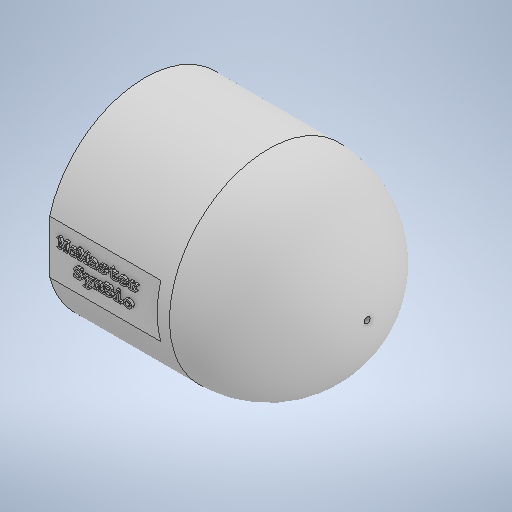
# Autodesk Inventor part: Bactria Membrane Half 1
Saved by Autodesk Inventor 2025 (Build 290162000, 162)
## iProperties
Created: 2024-08-12
Part Number: Bactria Membrane Half 1
Material: Generic
Document SubType Name: Modeling
Designer: kellst1
Density: 1 g/cm^3
Appearance: Default
Author: kellst1
Autodesk Inventor part; units mm, degrees
(part 1 of 2)
ref_plane "YZ Plane" through (0, 0, 0) normal (1, 0, 0) x (0, 1, 0)
ref_plane "XZ Plane" through (0, 0, 0) normal (0, 1, 0) x (-1, 0, 0)
ref_plane "XY Plane" through (0, 0, 0) normal (0, 0, 1) x (1, 0, 0)
sketch "Sketch1" plane through (0, 0, 0) normal (1, 0, 0) x (0, 1, 0)
  arc A0 (0, -80) -> (0, 80) centre (0, 0) ccw
  arc A1 (0, -65) -> (0, 65) centre (0, 0) ccw
  line L0 (0, 80) -> (0, -80)
  dimension "d0" = 160
  dimension "d1" = 130
  constraints: 4 point on circle, 2 centre point, 2 coincident, 2 end point, 2 point on line, 1 vertical
  measures "d0" diameter of A0
  measures "d1" diameter of A1
revolve "Revolution1" add sketch "Sketch1" angle 180 about axis through (0, 0, 80) along (0, 0, -1) contours L0 A1 A0
sketch "Sketch3" plane through (0, 0, 0) normal (-1, 0, 0) x (0, 0, 1)
  circle A0 centre (0, 0) radius 65
  circle A1 centre (0, 0) radius 80
  constraints: 2 centre point, 2 coincident
extrude "Extrusion2" add sketch "Sketch3" along normal blind 80
sketch "Sketch4" plane through (-80, 0, 0) normal (-1, 0, 0) x (0, 0, 1)
  circle A0 centre (0, 0) radius 72.5
  circle A1 centre (0, 0) radius 80
  dimension "d9" = 145
  dimension "d10" = 160
  constraints: 2 centre point, 1 coincident
  measures "d9" diameter of A0
  measures "d10" diameter of A1
extrude "Extrusion3" add sketch "Sketch4" along normal blind 20
thread "Thread2" size "M50x4" class "6H" standard "ANSI Metric M Profile" length 20
sketch "Sketch5" plane through (-100, 0, 0) normal (-1, 0, 0) x (0, 0, 1)
  circle A0 centre (0, 0) radius 2.5
  dimension "d15" = 5
  constraints: 1 centre point, 1 coincident
  measures "d15" diameter of A0
extrude "Extrusion4" cut sketch "Sketch5" against normal blind 200
sketch "Sketch7" plane through (-100, 0, 0) normal (-1, 0, 0) x (0, 0, 1)
  circle A0 centre (0, 0) radius 80 projected
  line L0 (77.0624, 21.48) -> (77.0624, -21.48)
  line L1 (77.0624, 21.48) -> (81.6145, 21.48)
  line L2 (81.6145, 21.48) -> (81.6145, -21.48)
  line L3 (81.6145, -21.48) -> (77.0624, -21.48)
  constraints: 8 end point, 2 perpendicular, 2 point on circle, 1 horizontal, 1 vertical
extrude "Extrusion5" cut sketch "Sketch7" against normal blind 90 contours A0 L0 picked at (77.6049, -4.8062)
sketch "Sketch8" plane through (-100, -21.48, 77.0624) normal (0, 0, 1) x (1, 0, 0)
  line L0 (1.6316, 42.4882) -> (87.8375, 42.4882) construction
  line L1 (87.8375, 42.4882) -> (87.8375, 0.6662) construction
  line L2 (87.8375, 0.6662) -> (1.6316, 0.6662) construction
  line L3 (1.6316, 0.6662) -> (1.6316, 42.4882) construction
  line L4 (10.2061, 31.2629) -> (10.2061, 27.2367)
  line L5 (10.2061, 27.2367) -> (10.6916, 27.2367)
  spline S0 degree 2 poles (10.6916, 27.2367) (11.1995, 27.2367) (11.6178, 26.8632) (11.6178, 26.557) knots 0 0 0 1 2 2 2
  spline S1 degree 2 poles (11.6178, 26.557) (11.6178, 26.2507) (11.1995, 25.8847) (10.6916, 25.8847) knots 0 0 0 1 2 2 2
  line L6 (10.6916, 25.8847) -> (8.8541, 25.8847)
  spline S2 degree 2 poles (8.8541, 25.8847) (8.3461, 25.8847) (7.9278, 26.2582) (7.9278, 26.5645) knots 0 0 0 1 2 2 2
  spline S3 degree 2 poles (7.9278, 26.5645) (7.9278, 26.8707) (8.3461, 27.2367) (8.8541, 27.2367) knots 0 0 0 1 2 2 2
  line L7 (8.8541, 27.2367) -> (8.8541, 32.5327)
  spline S4 degree 2 poles (8.8541, 32.5327) (8.3461, 32.5327) (7.9278, 32.9062) (7.9278, 33.2125) knots 0 0 0 1 2 2 2
  spline S5 degree 2 poles (7.9278, 33.2125) (7.9278, 33.5112) (8.3461, 33.8847) (8.8541, 33.8847) knots 0 0 0 1 2 2 2
  line L8 (8.8541, 33.8847) -> (10.5273, 33.8773)
  line L9 (10.5273, 33.8773) -> (12.3648, 29.8063)
  line L10 (12.3648, 29.8063) -> (14.1799, 33.8847)
  line L11 (14.1799, 33.8847) -> (15.8531, 33.8773)
  spline S6 degree 2 poles (15.8531, 33.8773) (16.3611, 33.8773) (16.7794, 33.5112) (16.7794, 33.205) knots 0 0 0 1 2 2 2
  spline S7 degree 2 poles (16.7794, 33.205) (16.7794, 32.8987) (16.3611, 32.5252) (15.8531, 32.5252) knots 0 0 0 1 2 2 2
  line L12 (15.8531, 32.5252) -> (15.8531, 27.2367)
  spline S8 degree 2 poles (15.8531, 27.2367) (16.3611, 27.2367) (16.7794, 26.8632) (16.7794, 26.557) knots 0 0 0 1 2 2 2
  spline S9 degree 2 poles (16.7794, 26.557) (16.7794, 26.2507) (16.3611, 25.8847) (15.8531, 25.8847) knots 0 0 0 1 2 2 2
  line L13 (15.8531, 25.8847) -> (14.0081, 25.8847)
  spline S10 degree 2 poles (14.0081, 25.8847) (13.5002, 25.8847) (13.0819, 26.2582) (13.0819, 26.5645) knots 0 0 0 1 2 2 2
  spline S11 degree 2 poles (13.0819, 26.5645) (13.0819, 26.8707) (13.5002, 27.2367) (14.0081, 27.2367) knots 0 0 0 1 2 2 2
  line L14 (14.0081, 27.2367) -> (14.5011, 27.2367)
  line L15 (14.5011, 27.2367) -> (14.5011, 31.2629)
  line L16 (14.5011, 31.2629) -> (12.9474, 27.782)
  line L17 (12.9474, 27.782) -> (11.7747, 27.782)
  line L18 (11.7747, 27.782) -> (10.2061, 31.2629)
  spline S12 degree 2 poles (22.531, 31.6214) (22.77, 31.8604) (23.0315, 31.8604) knots 0 0 0 1 1 1
  spline S13 degree 2 poles (23.0315, 31.8604) (23.3228, 31.8604) (23.6963, 31.4421) (23.6963, 30.9641) knots 0 0 0 1 2 2 2
  line L19 (23.6963, 30.9641) -> (23.6963, 30.0901)
  spline S14 degree 2 poles (23.6963, 30.0901) (23.6963, 29.6046) (23.3228, 29.1938) (23.0165, 29.1938) knots 0 0 0 1 2 2 2
  spline S15 degree 2 poles (23.0165, 29.1938) (22.7402, 29.1938) (22.546, 29.3506) knots 0 0 0 1 1 1
  spline S16 degree 2 poles (22.546, 29.3506) (22.4115, 29.4702) (22.2546, 30.2022) (21.9484, 30.3815) knots 0 0 0 1 2 2 2
  spline S17 degree 2 poles (21.9484, 30.3815) (21.418, 30.6952) (20.5814, 30.6952) knots 0 0 0 1 1 1
  spline S18 degree 2 poles (20.5814, 30.6952) (19.6253, 30.6952) (18.475, 29.5747) (18.475, 28.7232) knots 0 0 0 1 2 2 2
  spline S19 degree 2 poles (18.475, 28.7232) (18.475, 27.9314) (19.5805, 27.0201) (20.8653, 27.0201) knots 0 0 0 1 2 2 2
  spline S20 degree 2 poles (20.8653, 27.0201) (21.7094, 27.0201) (22.2472, 27.1919) knots 0 0 0 1 1 1
  spline S21 degree 2 poles (22.2472, 27.1919) (22.5609, 27.2965) (23.1286, 27.8044) (23.3601, 27.8044) knots 0 0 0 1 2 2 2
  spline S22 degree 2 poles (23.3601, 27.8044) (23.6365, 27.8044) (24.0399, 27.3936) (24.0399, 27.1172) knots 0 0 0 1 2 2 2
  spline S23 degree 2 poles (24.0399, 27.1172) (24.0399, 26.669) (23.4274, 26.2657) knots 0 0 0 1 1 1
  spline S24 degree 2 poles (23.4274, 26.2657) (22.5161, 25.6681) (20.7607, 25.6681) knots 0 0 0 1 1 1
  spline S25 degree 2 poles (20.7607, 25.6681) (19.1846, 25.6681) (18.3107, 26.318) knots 0 0 0 1 1 1
  spline S26 degree 2 poles (18.3107, 26.318) (17.123, 27.1919) (17.123, 28.7157) knots 0 0 0 1 1 1
  spline S27 degree 2 poles (17.123, 28.7157) (17.123, 30.1574) (19.0502, 32.0472) (20.5964, 32.0472) knots 0 0 0 1 2 2 2
  spline S28 degree 2 poles (20.5964, 32.0472) (21.1566, 32.0472) (22.1202, 31.838) (22.531, 31.6214) knots 0 0 0 1 2 2 2
  line L20 (26.4152, 31.2629) -> (26.4152, 27.2367)
  line L21 (26.4152, 27.2367) -> (26.9008, 27.2367)
  spline S29 degree 2 poles (26.9008, 27.2367) (27.4087, 27.2367) (27.827, 26.8632) (27.827, 26.557) knots 0 0 0 1 2 2 2
  spline S30 degree 2 poles (27.827, 26.557) (27.827, 26.2507) (27.4087, 25.8847) (26.9008, 25.8847) knots 0 0 0 1 2 2 2
  line L22 (26.9008, 25.8847) -> (25.0632, 25.8847)
  spline S31 degree 2 poles (25.0632, 25.8847) (24.5553, 25.8847) (24.137, 26.2582) (24.137, 26.5645) knots 0 0 0 1 2 2 2
  spline S32 degree 2 poles (24.137, 26.5645) (24.137, 26.8707) (24.5553, 27.2367) (25.0632, 27.2367) knots 0 0 0 1 2 2 2
  line L23 (25.0632, 27.2367) -> (25.0632, 32.5327)
  spline S33 degree 2 poles (25.0632, 32.5327) (24.5553, 32.5327) (24.137, 32.9062) (24.137, 33.2125) knots 0 0 0 1 2 2 2
  spline S34 degree 2 poles (24.137, 33.2125) (24.137, 33.5112) (24.5553, 33.8847) (25.0632, 33.8847) knots 0 0 0 1 2 2 2
  line L24 (25.0632, 33.8847) -> (26.7364, 33.8773)
  line L25 (26.7364, 33.8773) -> (28.574, 29.8063)
  line L26 (28.574, 29.8063) -> (30.3891, 33.8847)
  line L27 (30.3891, 33.8847) -> (32.0623, 33.8773)
  spline S35 degree 2 poles (32.0623, 33.8773) (32.5702, 33.8773) (32.9885, 33.5112) (32.9885, 33.205) knots 0 0 0 1 2 2 2
  spline S36 degree 2 poles (32.9885, 33.205) (32.9885, 32.8987) (32.5702, 32.5252) (32.0623, 32.5252) knots 0 0 0 1 2 2 2
  line L28 (32.0623, 32.5252) -> (32.0623, 27.2367)
  spline S37 degree 2 poles (32.0623, 27.2367) (32.5702, 27.2367) (32.9885, 26.8632) (32.9885, 26.557) knots 0 0 0 1 2 2 2
  spline S38 degree 2 poles (32.9885, 26.557) (32.9885, 26.2507) (32.5702, 25.8847) (32.0623, 25.8847) knots 0 0 0 1 2 2 2
  line L29 (32.0623, 25.8847) -> (30.2173, 25.8847)
  spline S39 degree 2 poles (30.2173, 25.8847) (29.7094, 25.8847) (29.291, 26.2582) (29.291, 26.5645) knots 0 0 0 1 2 2 2
  spline S40 degree 2 poles (29.291, 26.5645) (29.291, 26.8707) (29.7094, 27.2367) (30.2173, 27.2367) knots 0 0 0 1 2 2 2
  line L30 (30.2173, 27.2367) -> (30.7103, 27.2367)
  line L31 (30.7103, 27.2367) -> (30.7103, 31.2629)
  line L32 (30.7103, 31.2629) -> (29.1566, 27.782)
  line L33 (29.1566, 27.782) -> (27.9839, 27.782)
  line L34 (27.9839, 27.782) -> (26.4152, 31.2629)
  line L35 (37.8438, 25.8847) -> (37.8438, 26.1984)
  spline S41 degree 2 poles (37.8438, 26.1984) (37.3359, 25.937) (36.1108, 25.6681) (35.6104, 25.6681) knots 0 0 0 1 2 2 2
  spline S42 degree 2 poles (35.6104, 25.6681) (34.5273, 25.6681) (33.1678, 26.8184) (33.1678, 27.5131) knots 0 0 0 1 2 2 2
  spline S43 degree 2 poles (33.1678, 27.5131) (33.1678, 28.3646) (34.9008, 29.8138) (36.4246, 29.8138) knots 0 0 0 1 2 2 2
  spline S44 degree 2 poles (36.4246, 29.8138) (37.0371, 29.8138) (37.8438, 29.6793) knots 0 0 0 1 1 1
  line L36 (37.8438, 29.6793) -> (37.8438, 30.008)
  spline S45 degree 2 poles (37.8438, 30.008) (37.8438, 30.3142) (37.3209, 30.6952) (36.5964, 30.6952) knots 0 0 0 1 2 2 2
  spline S46 degree 2 poles (36.5964, 30.6952) (35.9913, 30.6952) (35.0352, 30.4562) knots 0 0 0 1 1 1
  spline S47 degree 2 poles (35.0352, 30.4562) (34.6841, 30.374) (34.4825, 30.374) knots 0 0 0 1 1 1
  spline S48 degree 2 poles (34.4825, 30.374) (34.2136, 30.374) (33.8401, 30.7624) (33.8401, 31.0687) knots 0 0 0 1 2 2 2
  spline S49 degree 2 poles (33.8401, 31.0687) (33.8401, 31.2405) (33.9745, 31.487) (34.2061, 31.6364) (34.587, 31.7409) knots 0 0 0 1 2 3 3 3
  spline S50 degree 2 poles (34.587, 31.7409) (35.0875, 31.8829) (36.1258, 32.0472) (36.5441, 32.0472) knots 0 0 0 1 2 2 2
  spline S51 degree 2 poles (36.5441, 32.0472) (37.8065, 32.0472) (39.1958, 30.9566) (39.1958, 30.0154) knots 0 0 0 1 2 2 2
  line L37 (39.1958, 30.0154) -> (39.1958, 27.2367)
  line L38 (39.1958, 27.2367) -> (39.4274, 27.2367)
  spline S52 degree 2 poles (39.4274, 27.2367) (39.9353, 27.2367) (40.3536, 26.8632) (40.3536, 26.557) knots 0 0 0 1 2 2 2
  spline S53 degree 2 poles (40.3536, 26.557) (40.3536, 26.2507) (39.9353, 25.8847) (39.4274, 25.8847) knots 0 0 0 1 2 2 2
  line L39 (39.4274, 25.8847) -> (37.8438, 25.8847)
  spline S54 degree 2 poles (37.8438, 28.3049) (37.0371, 28.4618) (36.3499, 28.4618) knots 0 0 0 1 1 1
  spline S55 degree 2 poles (36.3499, 28.4618) (35.5282, 28.4618) (34.9306, 28.0584) knots 0 0 0 1 1 1
  spline S56 degree 2 poles (34.9306, 28.0584) (34.5646, 27.8044) (34.5646, 27.543) knots 0 0 0 1 1 1
  spline S57 degree 2 poles (34.5646, 27.543) (34.5646, 27.3562) (34.7439, 27.2367) knots 0 0 0 1 1 1
  spline S58 degree 2 poles (34.7439, 27.2367) (35.0726, 27.0201) (35.6477, 27.0201) knots 0 0 0 1 1 1
  spline S59 degree 2 poles (35.6477, 27.0201) (36.1333, 27.0201) (37.3657, 27.4011) (37.8438, 27.7297) knots 0 0 0 1 2 2 2
  line L40 (37.8438, 27.7297) -> (37.8438, 28.3049)
  spline S60 degree 2 poles (46.1949, 30.2918) (45.8662, 30.4935) (45.1417, 30.6952) (44.7458, 30.6952) knots 0 0 0 1 2 2 2
  spline S61 degree 2 poles (44.7458, 30.6952) (43.9615, 30.6952) (43.4983, 30.4412) knots 0 0 0 1 1 1
  spline S62 degree 2 poles (43.4983, 30.4412) (43.2967, 30.3292) (43.2967, 30.1947) knots 0 0 0 1 1 1
  spline S63 degree 2 poles (43.2967, 30.1947) (43.2967, 30.0453) (43.573, 29.8959) knots 0 0 0 1 1 1
  spline S64 degree 2 poles (43.573, 29.8959) (43.7822, 29.7914) (44.5142, 29.6942) knots 0 0 0 1 1 1
  spline S65 degree 2 poles (44.5142, 29.6942) (45.8587, 29.5075) (46.3891, 29.3282) knots 0 0 0 1 1 1
  spline S66 degree 2 poles (46.3891, 29.3282) (47.0763, 29.0817) (47.8307, 28.1182) (47.8307, 27.5878) knots 0 0 0 1 2 2 2
  spline S67 degree 2 poles (47.8307, 27.5878) (47.8307, 26.8632) (47.1883, 26.3703) knots 0 0 0 1 1 1
  spline S68 degree 2 poles (47.1883, 26.3703) (46.277, 25.6681) (44.813, 25.6681) knots 0 0 0 1 1 1
  spline S69 degree 2 poles (44.813, 25.6681) (44.2229, 25.6681) (43.2294, 25.8698) (42.8186, 26.064) knots 0 0 0 1 2 2 2
  spline S70 degree 2 poles (42.8186, 26.064) (42.714, 25.9744) (42.4899, 25.8847) (42.3779, 25.8847) knots 0 0 0 1 2 2 2
  spline S71 degree 2 poles (42.3779, 25.8847) (42.0567, 25.8847) (41.6832, 26.303) (41.6832, 26.7886) knots 0 0 0 1 2 2 2
  line L41 (41.6832, 26.7886) -> (41.6832, 27.2442)
  spline S72 degree 2 poles (41.6832, 27.2442) (41.6832, 27.7297) (42.0567, 28.148) (42.3629, 28.148) knots 0 0 0 1 2 2 2
  spline S73 degree 2 poles (42.3629, 28.148) (42.602, 28.148) (42.9306, 27.8791) (43.0277, 27.5505) knots 0 0 0 1 2 2 2
  spline S74 degree 2 poles (43.0277, 27.5505) (43.334, 27.289) (44.208, 27.0201) (44.7682, 27.0201) knots 0 0 0 1 2 2 2
  spline S75 degree 2 poles (44.7682, 27.0201) (45.7019, 27.0201) (46.2098, 27.3114) knots 0 0 0 1 1 1
  spline S76 degree 2 poles (46.2098, 27.3114) (46.4563, 27.4534) (46.4563, 27.6102) knots 0 0 0 1 1 1
  spline S77 degree 2 poles (46.4563, 27.6102) (46.4563, 27.8791) (46.1052, 28.0509) knots 0 0 0 1 1 1
  spline S78 degree 2 poles (46.1052, 28.0509) (45.7616, 28.2153) (44.6636, 28.3348) knots 0 0 0 1 1 1
  spline S79 degree 2 poles (44.6636, 28.3348) (43.0427, 28.5066) (42.4899, 28.9996) knots 0 0 0 1 1 1
  spline S80 degree 2 poles (42.4899, 28.9996) (41.9446, 29.4776) (41.9446, 30.1798) knots 0 0 0 1 1 1
  spline S81 degree 2 poles (41.9446, 30.1798) (41.9446, 30.9043) (42.5572, 31.3899) knots 0 0 0 1 1 1
  spline S82 degree 2 poles (42.5572, 31.3899) (43.3863, 32.0472) (44.7308, 32.0472) knots 0 0 0 1 1 1
  spline S83 degree 2 poles (44.7308, 32.0472) (45.2014, 32.0472) (46.0604, 31.8754) (46.4563, 31.6886) knots 0 0 0 1 2 2 2
  spline S84 degree 2 poles (46.4563, 31.6886) (46.5833, 31.7858) (46.7999, 31.8754) (46.897, 31.8754) knots 0 0 0 1 2 2 2
  spline S85 degree 2 poles (46.897, 31.8754) (47.1734, 31.8754) (47.5394, 31.4571) (47.5394, 30.9716) knots 0 0 0 1 2 2 2
  line L42 (47.5394, 30.9716) -> (47.5394, 30.6429)
  spline S86 degree 2 poles (47.5394, 30.6429) (47.5394, 30.2022) (47.4348, 30.0453) knots 0 0 0 1 1 1
  spline S87 degree 2 poles (47.4348, 30.0453) (47.2257, 29.7391) (46.8597, 29.7391) knots 0 0 0 1 1 1
  spline S88 degree 2 poles (46.8597, 29.7391) (46.6132, 29.7391) (46.2472, 30.0379) (46.1949, 30.2918) knots 0 0 0 1 2 2 2
  line L43 (52.5067, 30.5234) -> (52.5067, 27.8119)
  spline S89 degree 2 poles (52.5067, 27.8119) (52.5067, 27.3787) (52.686, 27.2367) knots 0 0 0 1 1 1
  spline S90 degree 2 poles (52.686, 27.2367) (52.9624, 27.0201) (53.672, 27.0201) knots 0 0 0 1 1 1
  spline S91 degree 2 poles (53.672, 27.0201) (54.7103, 27.0201) (55.5842, 27.4608) knots 0 0 0 1 1 1
  spline S92 degree 2 poles (55.5842, 27.4608) (55.9204, 27.6326) (56.1146, 27.6326) knots 0 0 0 1 1 1
  spline S93 degree 2 poles (56.1146, 27.6326) (56.376, 27.6326) (56.7644, 27.2367) (56.7644, 26.9529) knots 0 0 0 1 2 2 2
  spline S94 degree 2 poles (56.7644, 26.9529) (56.7644, 26.6914) (56.5553, 26.4972) knots 0 0 0 1 1 1
  spline S95 degree 2 poles (56.5553, 26.4972) (56.2341, 26.191) (54.3219, 25.6681) (53.672, 25.6681) knots 0 0 0 1 2 2 2
  spline S96 degree 2 poles (53.672, 25.6681) (52.4171, 25.6681) (51.1547, 26.7587) (51.1547, 27.5505) knots 0 0 0 1 2 2 2
  line L44 (51.1547, 27.5505) -> (51.1547, 30.5234)
  line L45 (51.1547, 30.5234) -> (50.6692, 30.5234)
  spline S97 degree 2 poles (50.6692, 30.5234) (50.1837, 30.5234) (49.7654, 30.8969) (49.7654, 31.2031) knots 0 0 0 1 2 2 2
  spline S98 degree 2 poles (49.7654, 31.2031) (49.7654, 31.5019) (50.1837, 31.8754) (50.6692, 31.8754) knots 0 0 0 1 2 2 2
  line L46 (50.6692, 31.8754) -> (51.1547, 31.8754)
  line L47 (51.1547, 31.8754) -> (51.1547, 33.0929)
  spline S99 degree 2 poles (51.1547, 33.0929) (51.1547, 33.5785) (51.5282, 33.9968) (51.8345, 33.9968) knots 0 0 0 1 2 2 2
  spline S100 degree 2 poles (51.8345, 33.9968) (52.1333, 33.9968) (52.5067, 33.5785) (52.5067, 33.0929) knots 0 0 0 1 2 2 2
  line L48 (52.5067, 33.0929) -> (52.5067, 31.8754)
  line L49 (52.5067, 31.8754) -> (55.0016, 31.8754)
  spline S101 degree 2 poles (55.0016, 31.8754) (55.4871, 31.8754) (55.9054, 31.5019) (55.9054, 31.1956) knots 0 0 0 1 2 2 2
  spline S102 degree 2 poles (55.9054, 31.1956) (55.9054, 30.8969) (55.4871, 30.5234) (55.0016, 30.5234) knots 0 0 0 1 2 2 2
  line L50 (55.0016, 30.5234) -> (52.5067, 30.5234)
  line L51 (64.3387, 28.1928) -> (58.7887, 28.1928)
  spline S103 degree 2 poles (58.7887, 28.1928) (58.9979, 27.6625) (60.0735, 27.0201) (60.9923, 27.0201) knots 0 0 0 1 2 2 2
  spline S104 degree 2 poles (60.9923, 27.0201) (61.7467, 27.0201) (62.9941, 27.3413) knots 0 0 0 1 1 1
  spline S105 degree 2 poles (62.9941, 27.3413) (63.5095, 27.4758) (63.7037, 27.4758) knots 0 0 0 1 1 1
  spline S106 degree 2 poles (63.7037, 27.4758) (63.9801, 27.4758) (64.3461, 27.0948) (64.3461, 26.8035) knots 0 0 0 1 2 2 2
  spline S107 degree 2 poles (64.3461, 26.8035) (64.3461, 26.5421) (64.1519, 26.3553) knots 0 0 0 1 1 1
  spline S108 degree 2 poles (64.1519, 26.3553) (63.883, 26.1088) (61.8363, 25.6681) (60.8952, 25.6681) knots 0 0 0 1 2 2 2
  spline S109 degree 2 poles (60.8952, 25.6681) (59.2742, 25.6681) (57.3247, 27.4982) (57.3247, 28.8352) knots 0 0 0 1 2 2 2
  spline S110 degree 2 poles (57.3247, 28.8352) (57.3247, 30.2619) (59.4311, 32.0472) (60.8055, 32.0472) knots 0 0 0 1 2 2 2
  spline S111 degree 2 poles (60.8055, 32.0472) (61.6272, 32.0472) (63.0091, 31.4646) (63.3452, 31.1284) knots 0 0 0 1 2 2 2
  spline S112 degree 2 poles (63.3452, 31.1284) (63.8158, 30.6429) (64.1295, 29.9258) knots 0 0 0 1 1 1
  spline S113 degree 2 poles (64.1295, 29.9258) (64.3387, 29.4253) (64.3387, 28.768) knots 0 0 0 1 1 1
  line L52 (64.3387, 28.768) -> (64.3387, 28.1928)
  spline S114 degree 2 poles (62.8447, 29.5449) (62.531, 30.12) (61.5301, 30.6952) (60.8354, 30.6952) knots 0 0 0 1 2 2 2
  spline S115 degree 2 poles (60.8354, 30.6952) (60.1482, 30.6952) (59.1398, 30.12) (58.8261, 29.5449) knots 0 0 0 1 2 2 2
  line L53 (58.8261, 29.5449) -> (62.8447, 29.5449)
  line L54 (68.7682, 31.8754) -> (68.7682, 31.0238)
  spline S116 degree 2 poles (68.7682, 31.0238) (69.6197, 31.6364) (70.6057, 32.0472) (71.0315, 32.0472) knots 0 0 0 1 2 2 2
  spline S117 degree 2 poles (71.0315, 32.0472) (71.6888, 32.0472) (72.3088, 31.5617) knots 0 0 0 1 1 1
  spline S118 degree 2 poles (72.3088, 31.5617) (72.7346, 31.233) (72.7346, 30.8894) knots 0 0 0 1 1 1
  spline S119 degree 2 poles (72.7346, 30.8894) (72.7346, 30.5981) (72.3312, 30.1947) (72.0474, 30.1947) knots 0 0 0 1 2 2 2
  spline S120 degree 2 poles (72.0474, 30.1947) (71.8009, 30.1947) (71.2406, 30.6952) (71.024, 30.6952) knots 0 0 0 1 2 2 2
  spline S121 degree 2 poles (71.024, 30.6952) (70.7402, 30.6952) (69.6122, 29.9856) (68.7682, 29.2685) knots 0 0 0 1 2 2 2
  line L55 (68.7682, 29.2685) -> (68.7682, 27.2367)
  line L56 (68.7682, 27.2367) -> (70.6953, 27.2367)
  spline S122 degree 2 poles (70.6953, 27.2367) (71.2033, 27.2367) (71.6216, 26.8632) (71.6216, 26.557) knots 0 0 0 1 2 2 2
  spline S123 degree 2 poles (71.6216, 26.557) (71.6216, 26.2507) (71.2033, 25.8847) (70.6953, 25.8847) knots 0 0 0 1 2 2 2
  line L57 (70.6953, 25.8847) -> (66.6094, 25.8847)
  spline S124 degree 2 poles (66.6094, 25.8847) (66.1015, 25.8847) (65.6832, 26.2582) (65.6832, 26.5645) knots 0 0 0 1 2 2 2
  spline S125 degree 2 poles (65.6832, 26.5645) (65.6832, 26.8707) (66.1015, 27.2367) (66.6094, 27.2367) knots 0 0 0 1 2 2 2
  line L58 (66.6094, 27.2367) -> (67.4162, 27.2367)
  line L59 (67.4162, 27.2367) -> (67.4162, 30.5234)
  line L60 (67.4162, 30.5234) -> (66.9306, 30.5234)
  spline S126 degree 2 poles (66.9306, 30.5234) (66.4227, 30.5234) (66.0044, 30.8969) (66.0044, 31.2031) knots 0 0 0 1 2 2 2
  spline S127 degree 2 poles (66.0044, 31.2031) (66.0044, 31.5094) (66.4227, 31.8754) (66.9306, 31.8754) knots 0 0 0 1 2 2 2
  line L61 (66.9306, 31.8754) -> (68.7682, 31.8754)
  spline S128 degree 2 poles (22.4974, 12.3248) (22.3181, 12.1156) (22.1015, 11.9961) (21.9446, 11.9961) knots 0 0 0 1 2 2 2
  spline S129 degree 2 poles (21.9446, 11.9961) (21.6309, 11.9961) (21.2574, 12.4144) (21.2574, 12.8925) knots 0 0 0 1 2 2 2
  line L62 (21.2574, 12.8925) -> (21.2574, 13.8038)
  spline S130 degree 2 poles (21.2574, 13.8038) (21.2574, 14.2893) (21.6309, 14.7076) (21.9446, 14.7076) knots 0 0 0 1 2 2 2
  spline S131 degree 2 poles (21.9446, 14.7076) (22.1837, 14.7076) (22.5049, 14.4536) (22.6767, 13.871) (22.7663, 13.7664) knots 0 0 0 1 2 3 3 3
  spline S132 degree 2 poles (22.7663, 13.7664) (22.9605, 13.5573) (23.9316, 13.139) (24.5067, 13.139) knots 0 0 0 1 2 2 2
  spline S133 degree 2 poles (24.5067, 13.139) (25.4106, 13.139) (25.9932, 13.5573) knots 0 0 0 1 1 1
  spline S134 degree 2 poles (25.9932, 13.5573) (26.3592, 13.8187) (26.3592, 14.1922) knots 0 0 0 1 1 1
  spline S135 degree 2 poles (26.3592, 14.1922) (26.3592, 14.4462) (26.0081, 14.8869) (25.6048, 15.0288) knots 0 0 0 1 2 2 2
  spline S136 degree 2 poles (25.6048, 15.0288) (25.3433, 15.1259) (24.432, 15.2977) knots 0 0 0 1 1 1
  spline S137 degree 2 poles (24.432, 15.2977) (23.3265, 15.5068) (22.1911, 16.082) (21.5263, 17.1352) (21.5263, 17.7477) knots 0 0 0 1 2 3 3 3
  spline S138 degree 2 poles (21.5263, 17.7477) (21.5263, 18.7188) (23.1473, 20.1754) (24.447, 20.1754) knots 0 0 0 1 2 2 2
  spline S139 degree 2 poles (24.447, 20.1754) (24.9699, 20.1754) (25.8587, 19.9438) (26.2248, 19.7048) knots 0 0 0 1 2 2 2
  spline S140 degree 2 poles (26.2248, 19.7048) (26.4862, 19.9662) (26.7551, 19.9662) knots 0 0 0 1 1 1
  spline S141 degree 2 poles (26.7551, 19.9662) (27.0539, 19.9662) (27.4274, 19.5479) (27.4274, 19.0699) knots 0 0 0 1 2 2 2
  line L63 (27.4274, 19.0699) -> (27.4274, 18.054)
  spline S142 degree 2 poles (27.4274, 18.054) (27.4274, 17.5685) (27.0539, 17.1502) (26.7551, 17.1502) knots 0 0 0 1 2 2 2
  spline S143 degree 2 poles (26.7551, 17.1502) (26.5086, 17.1502) (26.3219, 17.2996) knots 0 0 0 1 1 1
  spline S144 degree 2 poles (26.3219, 17.2996) (26.1725, 17.4116) (26.0305, 18.0839) (25.9185, 18.2333) knots 0 0 0 1 2 2 2
  spline S145 degree 2 poles (25.9185, 18.2333) (25.7243, 18.4798) (24.9624, 18.8234) (24.4619, 18.8234) knots 0 0 0 1 2 2 2
  spline S146 degree 2 poles (24.4619, 18.8234) (23.7299, 18.8234) (22.8784, 18.1436) (22.8784, 17.7776) knots 0 0 0 1 2 2 2
  spline S147 degree 2 poles (22.8784, 17.7776) (22.8784, 17.5236) (23.2294, 17.0605) (23.5581, 16.9261) knots 0 0 0 1 2 2 2
  spline S148 degree 2 poles (23.5581, 16.9261) (23.7822, 16.8364) (25.8513, 16.4256) (26.9717, 15.9401) (27.7112, 14.8943) (27.7112, 14.1772) knots 0 0 0 1 2 3 4 4 4
  spline S149 degree 2 poles (27.7112, 14.1772) (27.7112, 13.1763) (27.0091, 12.5787) knots 0 0 0 1 1 1
  spline S150 degree 2 poles (27.0091, 12.5787) (26.0679, 11.787) (24.6188, 11.787) knots 0 0 0 1 1 1
  spline S151 degree 2 poles (24.6188, 11.787) (24.0586, 11.787) (22.9979, 12.0559) (22.4974, 12.3248) knots 0 0 0 1 2 2 2
  line L64 (31.827, 12.011) -> (29.4815, 16.6198)
  spline S152 degree 2 poles (29.4815, 16.6198) (28.9736, 16.6198) (28.5553, 16.9858) (28.5553, 17.2921) knots 0 0 0 1 2 2 2
  spline S153 degree 2 poles (28.5553, 17.2921) (28.5553, 17.5983) (28.9736, 17.9718) (29.4815, 17.9718) knots 0 0 0 1 2 2 2
  line L65 (29.4815, 17.9718) -> (30.9904, 17.9718)
  spline S154 degree 2 poles (30.9904, 17.9718) (31.4909, 17.9718) (31.9092, 17.5983) (31.9092, 17.2921) knots 0 0 0 1 2 2 2
  spline S155 degree 2 poles (31.9092, 17.2921) (31.9092, 16.9858) (31.4909, 16.6198) (30.9904, 16.6198) knots 0 0 0 1 2 2 2
  line L66 (30.9904, 16.6198) -> (32.5814, 13.4975)
  line L67 (32.5814, 13.4975) -> (34.165, 16.6198)
  spline S156 degree 2 poles (34.165, 16.6198) (33.6645, 16.6198) (33.2462, 16.9933) (33.2462, 17.2996) knots 0 0 0 1 2 2 2
  spline S157 degree 2 poles (33.2462, 17.2996) (33.2462, 17.6058) (33.6645, 17.9718) (34.165, 17.9718) knots 0 0 0 1 2 2 2
  line L68 (34.165, 17.9718) -> (35.6813, 17.9718)
  spline S158 degree 2 poles (35.6813, 17.9718) (36.1893, 17.9718) (36.6076, 17.5983) (36.6076, 17.2921) knots 0 0 0 1 2 2 2
  spline S159 degree 2 poles (36.6076, 17.2921) (36.6076, 16.9858) (36.1893, 16.6198) (35.6813, 16.6198) knots 0 0 0 1 2 2 2
  line L69 (35.6813, 16.6198) -> (32.5814, 10.5096)
  spline S160 degree 2 poles (32.5814, 10.5096) (33.0894, 10.5096) (33.5973, 10.5096) knots 0 0 0 1 1 1
  spline S161 degree 2 poles (33.5973, 10.5096) (34.0156, 10.1362) (34.0156, 9.8299) knots 0 0 0 1 1 1
  spline S162 degree 2 poles (34.0156, 9.8299) (34.0156, 9.5236) (33.5973, 9.1576) (33.0894, 9.1576) knots 0 0 0 1 2 2 2
  line L70 (33.0894, 9.1576) -> (29.7206, 9.1576)
  spline S163 degree 2 poles (29.7206, 9.1576) (29.2201, 9.1576) (28.8018, 9.5236) (28.8018, 9.8299) knots 0 0 0 1 2 2 2
  spline S164 degree 2 poles (28.8018, 9.8299) (28.8018, 10.1362) (29.2201, 10.5096) (29.7206, 10.5096) knots 0 0 0 1 2 2 2
  line L71 (29.7206, 10.5096) -> (31.0651, 10.5096)
  line L72 (31.0651, 10.5096) -> (31.827, 12.011)
  line L73 (39.3116, 17.9718) -> (39.3116, 17.5087)
  spline S165 degree 2 poles (39.3116, 17.5087) (39.6776, 17.8299) (40.574, 18.1436) (41.0894, 18.1436) knots 0 0 0 1 2 2 2
  spline S166 degree 2 poles (41.0894, 18.1436) (42.292, 18.1436) (42.9941, 17.3967) knots 0 0 0 1 1 1
  spline S167 degree 2 poles (42.9941, 17.3967) (43.5469, 16.8066) (43.5469, 15.843) knots 0 0 0 1 1 1
  line L74 (43.5469, 15.843) -> (43.5469, 13.3332)
  spline S168 degree 2 poles (43.5469, 13.3332) (44.0548, 13.3332) (44.4731, 12.9597) (44.4731, 12.6534) knots 0 0 0 1 2 2 2
  spline S169 degree 2 poles (44.4731, 12.6534) (44.4731, 12.3472) (44.0548, 11.9812) (43.5469, 11.9812) knots 0 0 0 1 2 2 2
  line L75 (43.5469, 11.9812) -> (42.1949, 11.9812)
  spline S170 degree 2 poles (42.1949, 11.9812) (41.6869, 11.9812) (41.2686, 12.3546) (41.2686, 12.6609) knots 0 0 0 1 2 2 2
  spline S171 degree 2 poles (41.2686, 12.6609) (41.2686, 12.9672) (41.6869, 13.3332) (42.1949, 13.3332) knots 0 0 0 1 2 2 2
  line L76 (42.1949, 13.3332) -> (42.1949, 15.8803)
  spline S172 degree 2 poles (42.1949, 15.8803) (42.1949, 16.321) (41.9558, 16.5302) knots 0 0 0 1 1 1
  spline S173 degree 2 poles (41.9558, 16.5302) (41.6496, 16.7916) (41.0296, 16.7916) knots 0 0 0 1 1 1
  spline S174 degree 2 poles (41.0296, 16.7916) (40.559, 16.7916) (39.8494, 16.4331) (39.3116, 15.843) knots 0 0 0 1 2 2 2
  line L77 (39.3116, 15.843) -> (39.3116, 13.3332)
  spline S175 degree 2 poles (39.3116, 13.3332) (39.8195, 13.3332) (39.954, 13.2062) knots 0 0 0 1 1 1
  spline S176 degree 2 poles (39.954, 13.2062) (40.2378, 12.9597) (40.2378, 12.6534) knots 0 0 0 1 1 1
  spline S177 degree 2 poles (40.2378, 12.6534) (40.2378, 12.3472) (39.8195, 11.9812) (39.3116, 11.9812) knots 0 0 0 1 2 2 2
  line L78 (39.3116, 11.9812) -> (37.9596, 11.9812)
  spline S178 degree 2 poles (37.9596, 11.9812) (37.4516, 11.9812) (37.0333, 12.3546) (37.0333, 12.6609) knots 0 0 0 1 2 2 2
  spline S179 degree 2 poles (37.0333, 12.6609) (37.0333, 12.9672) (37.3097, 13.2137) knots 0 0 0 1 1 1
  spline S180 degree 2 poles (37.3097, 13.2137) (37.4516, 13.3332) (37.9596, 13.3332) knots 0 0 0 1 1 1
  line L79 (37.9596, 13.3332) -> (37.9596, 16.6198)
  spline S181 degree 2 poles (37.9596, 16.6198) (37.4516, 16.6198) (37.0333, 16.9933) (37.0333, 17.2996) knots 0 0 0 1 2 2 2
  spline S182 degree 2 poles (37.0333, 17.2996) (37.0333, 17.6058) (37.4516, 17.9718) (37.9596, 17.9718) knots 0 0 0 1 2 2 2
  line L80 (37.9596, 17.9718) -> (39.3116, 17.9718)
  line L81 (46.0268, 13.3332) -> (46.0268, 18.6292)
  line L82 (46.0268, 18.6292) -> (45.8177, 18.6292)
  spline S183 degree 2 poles (45.8177, 18.6292) (45.3097, 18.6292) (44.8914, 19.0026) (44.8914, 19.3089) knots 0 0 0 1 2 2 2
  spline S184 degree 2 poles (44.8914, 19.3089) (44.8914, 19.6077) (45.3097, 19.9812) (45.8177, 19.9812) knots 0 0 0 1 2 2 2
  line L83 (45.8177, 19.9812) -> (49.2089, 19.9812)
  spline S185 degree 2 poles (49.2089, 19.9812) (50.419, 19.9812) (51.898, 18.6292) (51.898, 17.6955) knots 0 0 0 1 2 2 2
  spline S186 degree 2 poles (51.898, 17.6955) (51.898, 17.2547) (51.5544, 16.4704) (51.2108, 16.1418) knots 0 0 0 1 2 2 2
  spline S187 degree 2 poles (51.2108, 16.1418) (51.8531, 15.7608) (52.4881, 14.7375) (52.4881, 14.0951) knots 0 0 0 1 2 2 2
  spline S188 degree 2 poles (52.4881, 14.0951) (52.4881, 13.5797) (52.2565, 13.139) knots 0 0 0 1 1 1
  spline S189 degree 2 poles (52.2565, 13.139) (52.0847, 12.8028) (51.8382, 12.6086) knots 0 0 0 1 1 1
  spline S190 degree 2 poles (51.8382, 12.6086) (51.5021, 12.3322) (50.5235, 11.9812) (49.7915, 11.9812) knots 0 0 0 1 2 2 2
  line L84 (49.7915, 11.9812) -> (45.8177, 11.9812)
  spline S191 degree 2 poles (45.8177, 11.9812) (45.3097, 11.9812) (44.8914, 12.3546) (44.8914, 12.6609) knots 0 0 0 1 2 2 2
  spline S192 degree 2 poles (44.8914, 12.6609) (44.8914, 12.9672) (45.3097, 13.3332) (45.8177, 13.3332) knots 0 0 0 1 2 2 2
  line L85 (45.8177, 13.3332) -> (46.0268, 13.3332)
  line L86 (47.3788, 13.3332) -> (49.7168, 13.3332)
  spline S193 degree 2 poles (49.7168, 13.3332) (50.5385, 13.3332) (50.8821, 13.5797) knots 0 0 0 1 1 1
  spline S194 degree 2 poles (50.8821, 13.5797) (51.1361, 13.7589) (51.1361, 14.1025) knots 0 0 0 1 1 1
  spline S195 degree 2 poles (51.1361, 14.1025) (51.1361, 14.5059) (50.1202, 15.2977) (49.1715, 15.2977) knots 0 0 0 1 2 2 2
  line L87 (49.1715, 15.2977) -> (47.3788, 15.2977)
  line L88 (47.3788, 15.2977) -> (47.3788, 13.3332)
  line L89 (47.3788, 16.6497) -> (48.8653, 16.6497)
  spline S196 degree 2 poles (48.8653, 16.6497) (49.6645, 16.6497) (50.1874, 17.0531) knots 0 0 0 1 1 1
  spline S197 degree 2 poles (50.1874, 17.0531) (50.546, 17.3294) (50.546, 17.7328) knots 0 0 0 1 1 1
  spline S198 degree 2 poles (50.546, 17.7328) (50.546, 18.0913) (49.8737, 18.6292) (49.1417, 18.6292) knots 0 0 0 1 2 2 2
  line L90 (49.1417, 18.6292) -> (47.3788, 18.6292)
  line L91 (47.3788, 18.6292) -> (47.3788, 16.6497)
  line L92 (57.56, 17.9718) -> (57.56, 13.3332)
  line L93 (57.56, 13.3332) -> (59.1809, 13.3332)
  spline S199 degree 2 poles (59.1809, 13.3332) (59.6888, 13.3332) (60.1071, 12.9597) (60.1071, 12.6534) knots 0 0 0 1 2 2 2
  spline S200 degree 2 poles (60.1071, 12.6534) (60.1071, 12.3472) (59.6888, 11.9812) (59.1809, 11.9812) knots 0 0 0 1 2 2 2
  line L94 (59.1809, 11.9812) -> (54.587, 11.9812)
  spline S201 degree 2 poles (54.587, 11.9812) (54.0791, 11.9812) (53.6608, 12.3546) (53.6608, 12.6609) knots 0 0 0 1 2 2 2
  spline S202 degree 2 poles (53.6608, 12.6609) (53.6608, 12.9672) (54.0791, 13.3332) (54.587, 13.3332) knots 0 0 0 1 2 2 2
  line L95 (54.587, 13.3332) -> (56.208, 13.3332)
  line L96 (56.208, 13.3332) -> (56.208, 16.6198)
  line L97 (56.208, 16.6198) -> (55.1174, 16.6198)
  spline S203 degree 2 poles (55.1174, 16.6198) (54.6094, 16.6198) (54.1911, 16.9933) (54.1911, 17.2996) knots 0 0 0 1 2 2 2
  spline S204 degree 2 poles (54.1911, 17.2996) (54.1911, 17.6058) (54.6094, 17.9718) (55.1174, 17.9718) knots 0 0 0 1 2 2 2
  line L98 (55.1174, 17.9718) -> (57.56, 17.9718)
  line L99 (57.3732, 20.5339) -> (57.3732, 19.0997)
  line L100 (57.3732, 19.0997) -> (55.7672, 19.0997)
  line L101 (55.7672, 19.0997) -> (55.7672, 20.5339)
  line L102 (55.7672, 20.5339) -> (57.3732, 20.5339)
  spline S205 degree 2 poles (68.5105, 14.8645) (68.5105, 14.0876) (67.644, 12.631) (65.9409, 11.7645) (65.0072, 11.7645) knots 0 0 0 1 2 3 3 3
  spline S206 degree 2 poles (65.0072, 11.7645) (64.081, 11.7645) (62.3928, 12.6161) (61.5114, 14.0801) (61.5114, 14.8719) knots 0 0 0 1 2 3 3 3
  spline S207 degree 2 poles (61.5114, 14.8719) (61.5114, 15.6861) (62.4078, 17.2473) (64.0884, 18.1436) (65.0072, 18.1436) knots 0 0 0 1 2 3 3 3
  spline S208 degree 2 poles (65.0072, 18.1436) (65.9334, 18.1436) (67.6365, 17.2249) (68.5105, 15.6786) (68.5105, 14.8645) knots 0 0 0 1 2 3 3 3
  spline S209 degree 2 poles (67.1585, 14.857) (67.1585, 15.5068) (66.6879, 16.0521) knots 0 0 0 1 1 1
  spline S210 degree 2 poles (66.6879, 16.0521) (66.053, 16.7916) (65.0072, 16.7916) knots 0 0 0 1 1 1
  spline S211 degree 2 poles (65.0072, 16.7916) (64.0884, 16.7916) (62.8634, 15.6189) (62.8634, 14.8495) knots 0 0 0 1 2 2 2
  spline S212 degree 2 poles (62.8634, 14.8495) (62.8634, 14.2146) (64.1034, 13.1166) (65.0072, 13.1166) knots 0 0 0 1 2 2 2
  spline S213 degree 2 poles (65.0072, 13.1166) (65.9185, 13.1166) (67.1585, 14.2146) (67.1585, 14.857) knots 0 0 0 1 2 2 2
  point P0 (100, 21.48)
  constraints: 2 other
extrude "Extrusion6" add sketch "Sketch8" along normal blind 2
mirror "Mirror2" about plane through (0, 0, 0) normal (0, 0, 1) of "Extrusion5"